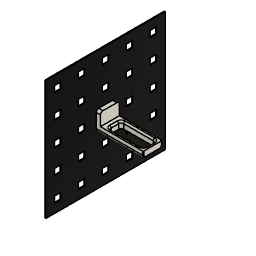
ParametricCrimperHolder (Autodesk Fusion 360 design; units mm, degrees)
Autodesk Fusion 360 part; units mm, degrees
sketch "Sketch1" plane through (0, 0, 0) normal (1, 0, 0) x (0, 1, 0) in component "Pegboard"
  line L0 (-95, 95) -> (95, 95)
  line L1 (95, 95) -> (95, -95)
  line L2 (95, -95) -> (-95, -95)
  line L3 (-95, -95) -> (-95, 95)
  dimension "d47" = 190
  dimension "d48" = 190
  dimension "d51" = 95
  dimension "d52" = 95
  constraint horizontal L0
  constraint vertical L1
  constraint horizontal L2
  constraint vertical L3
  measures "d47" distance of L0.start L0.end
  measures "d48" distance of L0.start L2.end
  measures "d51" distance of origin L0
  measures "d52" distance of origin L3
extrude "Extrude1" add sketch "Sketch1" against normal blind 1.2 makes body 1 in component "Pegboard"
ref_plane "WorkPlane1" through (0, -5, 0) normal (0, 1, 0) x (0, 0, 1) in component "HookPlate"
sketch "Sketch1 (2)" plane through (0, -5, 0) normal (0, 1, 0) x (1, 0, 0) in component "HookPlate"
  line L0 (-3.5, 10.6) -> (-1.5, 10.6)
  line L1 (-3.5, 10.6) -> (-3.5, 1.2)
  line L2 (-3.5, 1.2) -> (0.3, 1.2)
  line L3 (0.3, 1.2) -> (0.3, 4.7)
  line L4 (0.3, 4.7) -> (-1.5, 4.7)
  line L5 (-1.5, 10.6) -> (-1.5, 4.7)
  line L6 (0, 5) -> (-1.2, 5) construction
  line L7 (-1.2, 5) -> (-1.2, -5) construction
  line L8 (-1.2, -5) -> (0, -5) construction
  line L9 (0, -5) -> (0, 5) construction
  dimension "d28" = 2
  dimension "d61" = 1.2
  dimension "d62" = 10
  dimension "d63" = 5
  dimension "d68" = 9.4
  dimension "d69" = 0.3
  dimension "d70" = 0.3
  dimension "d71" = 3.5
  dimension "d72" = 0.3
  constraint perpendicular L0 L1
  constraint perpendicular L1 L2
  constraint perpendicular L3 L4
  constraint vertical L5
  constraint horizontal L6
  constraint vertical L7
  constraint horizontal L8
  constraint vertical L9
  constraint coincident origin L9
  constraint horizontal L2
  constraint vertical L3
  measures "d28" distance of L1 L4.end
  measures "d61" distance of L6.start L6.end
  measures "d62" distance of L6.start L8.end
  measures "d63" distance of origin L6
  measures "d68" distance of L0.start L1.end
  measures "d69" distance of L4 L6.end
  measures "d70" distance of L5 L6.end
  measures "d71" distance of L2.end L3.end
  measures "d72" distance of L3 L9
extrude "Extrude1'" add sketch "Sketch1 (2)" along normal blind 9.4 from surface at 0.3 separate body makes body 2 in component "HookPlate"
chamfer "Chamfer1" distance 1.5 angle 45 4 edges at (-2.5, 4.7, -10.6) (-2.5, -4.7, -10.6) (-1.6, 4.7, -1.2) (-1.6, -4.7, -1.2) on bodies 2 in component "HookPlate"
sketch "Sketch2" plane through (0, 0, 0) normal (1, 0, 0) x (0, 1, 0) in component "HookPlate"
  line L0 (19, -19) -> (-19, -19)
  line L1 (-19, -19) -> (-19, 19)
  line L2 (-19, 19) -> (19, 19)
  line L3 (19, 19) -> (19, -19)
  line L4 (19, -19) -> (-19, 19) construction
  line L5 (-19, -19) -> (19, 19) construction
  dimension "d23" = 38
  dimension "d24" = 38
  constraint horizontal L0
  constraint perpendicular L0 L1
  constraint parallel L0 L2
  constraint parallel L1 L3
  constraint coincident L4 origin
  constraint coincident L5 origin
  measures "d23" distance of L1.end L2.end
  measures "d24" distance of L0.end L1.end
extrude "Extrude2" add sketch "Sketch2" along normal blind 0.3 and the other way blind 10 separate body makes body 3 in component "HookPlate"
combine "Combine1" operation cut target body 3 tool bodies 2 in component "HookPlate"
sketch "Sketch3" plane through (0, 0, 0) normal (1, 0, 0) x (0, 1, 0) in component "HookPlate"
  line L0 (-19, 19) -> (19, 19)
  line L1 (19, 19) -> (19, -19)
  line L2 (19, -19) -> (-19, -19)
  line L3 (-19, -19) -> (-19, 19)
  dimension "d35" = 38
  dimension "d36" = 38
  dimension "d37" = 19
  dimension "d38" = 19
  constraint horizontal L0
  constraint vertical L1
  constraint horizontal L2
  constraint vertical L3
  measures "d35" distance of L0.start L0.end
  measures "d36" distance of L0.start L2.end
  measures "d37" horizontal distance of origin L0.start
  measures "d38" vertical distance of origin L0.start
extrude "Extrude3" add sketch "Sketch3" along normal blind 2 and the other way blind 10 separate body makes body 4 in component "HookPlate"
combine "Combine2" operation cut target body 4 tool bodies 3 keep tools in component "HookPlate"
pattern_linear "R-Pattern1" count 1 spacing 38 along (0, 1, 0) of "Combine2" in component "HookPlate"
sketch "Sketch4" plane through (0, 0, 0) normal (1, 0, 0) x (0, 1, 0) in component "HookPlate"
  line L0 (-11, 15) -> (11, 15)
  line L1 (15, 11) -> (15, -11)
  line L2 (11, -15) -> (-11, -15)
  line L3 (-15, -11) -> (-15, 11)
  arc A0 (-11, 15) -> (-15, 11) centre (-11, 11) ccw
  arc A1 (15, 11) -> (11, 15) centre (11, 11) ccw
  arc A2 (11, -15) -> (15, -11) centre (11, -11) ccw
  arc A3 (-15, -11) -> (-11, -15) centre (-11, -11) ccw
  line L4 (-19, 19) -> (19, 19)
  line L5 (19, 19) -> (19, -19)
  line L6 (19, -19) -> (-19, -19)
  line L7 (-19, -19) -> (-19, 19)
  point P0 (-15, 15)
  point P1 (15, 15)
  point P2 (-15, -15)
  dimension "d74" = 30
  dimension "d75" = 30
  dimension "d76" = 15
  dimension "d77" = 15
  dimension "d78" = 4
  dimension "d79" = 38
  dimension "d80" = 38
  dimension "d81" = 19
  dimension "d82" = 19
  constraint horizontal L0
  constraint vertical L1
  constraint horizontal L2
  constraint vertical L3
  constraint coincident P0 L3
  constraint coincident P0 L0
  constraint tangent L3 A0
  constraint tangent L0 A0
  constraint coincident P1 L0
  constraint coincident P1 L1
  constraint tangent L0 A1
  constraint tangent L1 A1
  constraint equal A0 A1
  constraint tangent L1 A2
  constraint tangent L2 A2
  constraint equal A0 A2
  constraint coincident P2 L2
  constraint coincident P2 L3
  constraint tangent L2 A3
  constraint tangent L3 A3
  constraint equal A0 A3
  constraint horizontal L4
  constraint vertical L5
  constraint horizontal L6
  constraint vertical L7
  measures "d74" distance of P0 P1
  measures "d75" distance of P0 P2
  measures "d76" distance of origin L0
  measures "d77" distance of origin L3
  measures "d78" radius of A0
  measures "d79" distance of L4.start L4.end
  measures "d80" distance of L4.start L6.end
  measures "d81" horizontal distance of origin L4.start
  measures "d82" distance of origin L4
extrude "Extrude4" cut sketch "Sketch4" along normal blind 100 bodies 4 in component "HookPlate"
sketch "Sketch2 (2)" plane through (0, 0, 0) normal (1, 0, 0) x (0, 1, 0) in component "Pegboard"
  line L0 (-95, 95) -> (-57, 95) construction
  line L1 (-57, 95) -> (-57, 57) construction
  line L2 (-57, 57) -> (-95, 57) construction
  line L3 (-95, 57) -> (-95, 95) construction
  line L4 (-81, 81) -> (-71, 81)
  line L5 (-71, 81) -> (-71, 71)
  line L6 (-71, 71) -> (-81, 71)
  line L7 (-81, 71) -> (-81, 81)
  dimension "d89" = 38
  dimension "d90" = 38
  dimension "d91" = 10
  dimension "d92" = 10
  dimension "d93" = 14
  dimension "d94" = 14
  dimension "d95" = 95
  dimension "d96" = 95
  constraint horizontal L0
  constraint vertical L1
  constraint horizontal L2
  constraint vertical L3
  constraint horizontal L4
  constraint vertical L5
  constraint horizontal L6
  constraint vertical L7
  measures "d89" distance of L0.start L0.end
  measures "d90" distance of L0.start L2.end
  measures "d91" distance of L4.start L4.end
  measures "d92" distance of L4.start L6.end
  measures "d93" distance of L3 L7
  measures "d94" distance of L0 L4
  measures "d95" distance of origin L0
  measures "d96" distance of origin L3
extrude "Extrude2'" add sketch "Sketch2 (2)" against normal blind 1.2 separate body makes body 5 in component "Pegboard"
combine "Combine1'" operation cut target body 1 tool bodies 5 in component "Pegboard"
pattern_linear "R-Pattern1'" count 5 spacing 38 along (0, 1, 0) count 5 spacing 38 along (0, 0, -1) of "Combine1'" in component "Pegboard"
sketch "Sketch1 (3)" plane through (2, 0, 0) normal (1, 0, 0) x (0, 1, 0) in component "PliersHolder"
  line L0 (-15, 11) -> (-15, -11)
  arc A0 (-15, -11) -> (-11, -15) centre (-11, -11) ccw
  line L1 (-11, -15) -> (11, -15)
  arc A1 (11, -15) -> (15, -11) centre (11, -11) ccw
  line L2 (15, -11) -> (15, 11)
  arc A2 (15, 11) -> (11, 15) centre (11, 11) ccw
  line L3 (11, 15) -> (-11, 15)
  arc A3 (-11, 15) -> (-15, 11) centre (-11, 11) ccw
extrude "Extrude1''" add sketch "Sketch1 (3)" along normal blind 5 separate body makes body 6 in component "PliersHolder"
sketch "Sketch2 (3)" plane through (7, 0, 0) normal (1, 0, 0) x (0, 1, 0) in component "PliersHolder"
  arc A0 (-11, 15) -> (-15, 11) centre (-11, 11) ccw construction
  line L0 (-15, 11) -> (-15, -11) construction
  arc A1 (-15, -11) -> (-11, -15) centre (-11, -11) ccw
  line L1 (-11, -15) -> (11, -15)
  arc A2 (11, -15) -> (15, -11) centre (11, -11) ccw
  line L2 (15, -11) -> (15, 11) construction
  arc A3 (15, 11) -> (11, 15) centre (11, 11) ccw construction
  line L3 (11, 15) -> (-11, 15) construction
  line L4 (-15, -5) -> (15, -5)
  line L5 (-15, -5) -> (-15, -11)
  line L6 (15, -5) -> (15, -11)
  dimension "d3" = 10
  constraint coincident L0 L4.start
  constraint coincident L2 L4.end
  constraint perpendicular L2 L4
  constraint coincident L0.end A1.start
  constraint coincident A2.end L2.start
  measures "d3" distance of L1 L4
extrude "Extrude2''" add sketch "Sketch2 (3)" along normal blind 68 bodies 6 in component "PliersHolder"
sketch "Sketch3 (2)" plane through (0, 0, -5) normal (0, 0, 1) x (-1, 0, 0) in component "PliersHolder"
  line L0 (-15, 10) -> (-70, 10)
  line L1 (-70, 10) -> (-70, -10)
  line L2 (-70, -10) -> (-15, -10)
  line L3 (-15, -10) -> (-15, 10)
  line L4 (-7, -15) -> (-7, 15) construction
  line L5 (-7, 15) -> (-75, 15) construction
  line L6 (-75, -15) -> (-7, -15) construction
  line L7 (-75, 15) -> (-75, -15) construction
  line L8 (-75, 0) -> (-7, 0) construction
  line L9 (-75, 0) -> (-7, 0) construction
  dimension "d6" = 55
  dimension "d7" = 20
  dimension "d16" = 30
  dimension "d56" = 5
  constraint horizontal L0
  constraint vertical L1
  constraint horizontal L2
  constraint vertical L3
  constraint coincident L5.end L7.start
  constraint coincident L6.start L7.end
  constraint midpoint L7 L8.start
  constraint midpoint L4 L8.end
  constraint symmetric L0 L2 L8
  measures "d6" distance of L0.start L0.end
  measures "d7" distance of L0.start L2.end
  measures "d16" distance of L5.end L6.start
  measures "d56" distance of L1 L5.end
extrude "Extrude3'" cut sketch "Sketch3 (2)" against normal blind 10 bodies 6 in component "PliersHolder"
fillet "Fillet1" radius 4 4 edges at (15, -10, -10) (15, 10, -10) (70, 10, -10) (70, -10, -10) on bodies 6 in component "PliersHolder"
fillet "Fillet2" radius 2.5 8 edges at (68.8284, 8.8284, -5) (42.5, 10, -5) (16.1716, 8.8284, -5) (15, 0, -5) (16.1716, -8.8284, -5) (42.5, -10, -5) (68.8284, -8.8284, -5) (70, 0, -5) on bodies 6 in component "PliersHolder"
fillet "Fillet3" radius 1 5 edges at (75, -15, -8) (75, -13.8284, -13.8284) (75, 0, -15) (75, 13.8284, -13.8284) (75, 15, -8) on bodies 6 in component "PliersHolder"
combine "Combine1''" [suppressed] in component "PliersHolder"
combine "Combine3" operation add target body 4 tool bodies 6 in component "HookPlate"
component "Base v2" placed x (1, 0, 0) y (0, 1, 0) z (0, 0, 1) at (0, 0, 0)
component "PliersHolder" placed x (1, 0, 0) y (0, 1, 0) z (0, 0, 1) at (0, 0, 0)
component "Pegboard" placed x (1, 0, 0) y (0, 1, 0) z (0, 0, 1) at (0, 0, 0) in component "Base v2"
component "HookPlate" placed x (1, 0, 0) y (0, 1, 0) z (0, 0, 1) at (0, 0, 0) in component "Base v2"
hidden bodies 3
equation "clearance = 0.3 mm"
equation "d18 = clearance"
equation "d19 = 10 mm - clearance * 2"
equation "width = 1"
equation "height = 1"
equation "d31 = clearance"
equation "d35 = ( 38 * width ) * 1 mm"
equation "d36 = ( 38 * height ) * 1 mm"
equation "d37 = ( 38 / 2 ) * 1 mm"
equation "d38 = ( 38 / 2 ) * 1 mm"
equation "d43 = width"
equation "d44 = height"
equation "d47 = ( 38 * ( width + 4 ) ) * 1 mm"
equation "d48 = ( 38 * ( height + 4 ) ) * 1 mm"
equation "d51 = ( 38 * 2.5 ) * 1 mm"
equation "d52 = d51"
equation "d68 = 10 mm - clearance * 2"
equation "d69 = clearance"
equation "d70 = clearance"
equation "d72 = clearance"
equation "inset = 4 mm"
equation "d74 = ( 38 * width ) * 1 mm - inset * 2"
equation "d75 = ( 38 * height ) * 1 mm - inset * 2"
equation "d76 = ( 38 / 2 ) * 1 mm - inset"
equation "d77 = ( 38 / 2 ) * 1 mm - inset"
equation "d79 = ( 38 * width ) * 1 mm"
equation "d80 = ( 38 * height ) * 1 mm"
equation "d81 = ( 38 / 2 ) * 1 mm"
equation "d82 = ( 38 / 2 ) * 1 mm"
equation "d93 = ( 38 / 2 ) * 1 mm - 5 mm"
equation "d94 = d93"
equation "d95 = ( 38 * 2.5 ) * 1 mm"
equation "d96 = d95"
equation "d99 = width + 4"
equation "d100 = height + 4"
equation "d4 = 68 mm - 55 mm + holeDepth"
equation "d6 = holeDepth"
equation "d7 = holeWidth"
equation "holeDepth = 55 mm"
equation "holeWidth = 20 mm"
